Autodesk Fusion 360 part; units mm, degrees
note: some values were not read from the file. Chosen so that the rebuilt part matches the saved one: which bodies a step acts on; which face or edge a step refers to. Set by a fixed rule: which sketch regions a step uses.
(part 4 of 4)
sketch "Base" plane through (0, 0, 52) normal (0, 0, 1) x (-1, 0, 0) in component "GPS"
  circle A0 centre (42.25, -34) radius 1.5
  circle A1 centre (-28.4, 34) radius 1.5
  circle A2 centre (-69.85, 16) radius 1.5
  arc A3 (32.5282, -1.6218) -> (32.5282, 1.6218) centre (30.9065, 0) ccw
  line L0 (32.5282, -1.6218) -> (14.9, -19.25)
  line L1 (14.9, -19.25) -> (7.5026, -19.25)
  arc A4 (5.6636, -14.8105) -> (7.5026, -19.25) centre (7.5026, -16.6494) ccw
  line L2 (5.6636, -14.8105) -> (18.5125, -1.9617)
  arc A5 (18.5125, -1.9617) -> (18.5125, 1.9617) centre (16.5508, 0) ccw
  line L3 (18.5125, 1.9617) -> (5.6636, 14.8105)
  arc A6 (7.5026, 19.25) -> (5.6636, 14.8105) centre (7.5026, 16.6494) ccw
  line L4 (7.5026, 19.25) -> (14.9, 19.25)
  line L5 (14.9, 19.25) -> (32.5282, 1.6218)
  circle A7 centre (-37.85, 16) radius 1.5
  arc A8 (3.4193, -1.5227) -> (3.4193, 1.5227) centre (1.8966, 0) ccw
  line L6 (3.4193, -1.5227) -> (-13.4941, -18.4361)
  spline S0 degree 5 poles (-13.4941, -18.4361) (-13.5655, -18.5075) (-13.7132, -18.651) (-13.9496, -18.869) (-14.3035, -19.15) (-14.8512, -19.4045) (-15.5396, -19.4698) (-16.3722, -19.2715) (-17.2898, -18.7896) (-18.1939, -18.0372) (-18.9671, -17.0431) (-19.3888, -16.0795) (-19.5532, -15.2733) (-19.5897, -14.7) (-19.5897, -14.4044) knots 0 0 0 0 0 0 0.1 0.2 0.3 0.4 0.5 0.6 0.7 0.8 0.9 1 1 1 1 1 1
  line L7 (-19.5897, -14.4044) -> (-19.5897, 14.4044)
  spline S1 degree 5 poles (-19.5897, 14.4044) (-19.5897, 14.7) (-19.5532, 15.2733) (-19.3888, 16.0795) (-18.9671, 17.0431) (-18.1939, 18.0372) (-17.2898, 18.7896) (-16.3722, 19.2715) (-15.5396, 19.4698) (-14.8512, 19.4045) (-14.3035, 19.15) (-13.9496, 18.869) (-13.7132, 18.651) (-13.5655, 18.5075) (-13.4941, 18.4361) knots -1 -1 -1 -1 -1 -1 -0.9 -0.8 -0.7 -0.6 -0.5 -0.4 -0.3 -0.2 -0.1 0 0 0 0 0 0
  line L8 (-13.4941, 18.4361) -> (3.4193, 1.5227)
  circle A9 centre (-28.4, -34) radius 1.5
  circle A10 centre (50.25, -29.25) radius 4
  circle A11 centre (-37.85, -16) radius 1.5
  circle A12 centre (-69.85, -16) radius 1.5
  line L9 (-8, -24.75) -> (24.8, -24.75)
  line L10 (24.8, -24.75) -> (27.0868, -27.0368)
  arc A13 (26.2737, -29) -> (27.0868, -27.0368) centre (26.2737, -27.85) ccw
  line L11 (26.2737, -29) -> (-9.4737, -29)
  arc A14 (-10.2868, -27.0368) -> (-9.4737, -29) centre (-9.4737, -27.85) ccw
  line L12 (-10.2868, -27.0368) -> (-8, -24.75)
  line L13 (27.0868, 27.0368) -> (24.8, 24.75)
  line L14 (24.8, 24.75) -> (-8, 24.75)
  line L15 (-8, 24.75) -> (-10.2868, 27.0368)
  arc A15 (-9.4737, 29) -> (-10.2868, 27.0368) centre (-9.4737, 27.85) ccw
  line L16 (-9.4737, 29) -> (26.2737, 29)
  arc A16 (27.0868, 27.0368) -> (26.2737, 29) centre (26.2737, 27.85) ccw
  line L17 (56.2, 11.1318) -> (56.2, -11.1318)
  arc A17 (55.4036, -12.729) -> (56.2, -11.1318) centre (54.2, -11.1318) ccw
  line L18 (55.4036, -12.729) -> (46.75, -19.25)
  line L19 (46.75, -19.25) -> (36.9216, -19.25)
  arc A18 (34.9726, -14.5445) -> (36.9216, -19.25) centre (36.9216, -16.4936) ccw
  line L20 (34.9726, -14.5445) -> (47.8662, -1.6509)
  arc A19 (47.8662, -1.6509) -> (47.8662, 1.6509) centre (46.2153, 0) ccw
  line L21 (47.8662, 1.6509) -> (34.9726, 14.5445)
  arc A20 (36.9216, 19.25) -> (34.9726, 14.5445) centre (36.9216, 16.4936) ccw
  line L22 (36.9216, 19.25) -> (46.75, 19.25)
  line L23 (46.75, 19.25) -> (55.4036, 12.729)
  arc A21 (56.2, 11.1318) -> (55.4036, 12.729) centre (54.2, 11.1318) ccw
  circle A22 centre (42.25, 34) radius 1.5
  line L24 (70.5, -12.5) -> (70.5, 12.5)
  line L25 (70.5, 12.5) -> (54.7221, 33.4587)
  arc A23 (54.7221, 33.4587) -> (52.2059, 35.2279) centre (50.7275, 30.4515) ccw
  line L26 (52.2059, 35.2279) -> (43.25, 38)
  line L27 (43.25, 38) -> (31.65, 38)
  line L28 (31.65, 38) -> (27.15, 33.5)
  line L29 (27.15, 33.5) -> (-9.25, 33.5)
  line L30 (-9.25, 33.5) -> (-13.75, 38)
  line L31 (-13.75, 38) -> (-30, 38)
  line L32 (-30, 38) -> (-42, 26.25)
  line L33 (-42, 26.25) -> (-70.822, 21.4463)
  arc A24 (-70.822, 21.4463) -> (-75, 16.5144) centre (-70, 16.5144) ccw
  line L34 (-75, 16.5144) -> (-75, -16.5144)
  arc A25 (-75, -16.5144) -> (-70.822, -21.4463) centre (-70, -16.5144) ccw
  line L35 (-70.822, -21.4463) -> (-42, -26.25)
  line L36 (-42, -26.25) -> (-30, -38)
  line L37 (-30, -38) -> (-13.75, -38)
  line L38 (-13.75, -38) -> (-9.25, -33.5)
  line L39 (-9.25, -33.5) -> (27.15, -33.5)
  line L40 (27.15, -33.5) -> (31.65, -38)
  line L41 (31.65, -38) -> (43.25, -38)
  line L42 (43.25, -38) -> (52.2059, -35.2279)
  arc A26 (52.2059, -35.2279) -> (54.7221, -33.4587) centre (50.7275, -30.4515) ccw
  line L43 (54.7221, -33.4587) -> (70.5, -12.5)
  line L44 (-37.85, -16) -> (-69.85, 16) construction
  line L45 (-69.85, -16) -> (-37.85, 16) construction
  arc A27 (-44.4808, -13.9654) -> (-39.8846, -9.3692) centre (-42.1827, -11.6673) ccw
  arc A28 (-67.8154, -9.3692) -> (-63.2192, -13.9654) centre (-65.5173, -11.6673) ccw
  arc A29 (-63.2192, 13.9654) -> (-67.8154, 9.3692) centre (-65.5173, 11.6673) ccw
  arc A30 (-39.8846, 9.3692) -> (-44.4808, 13.9654) centre (-42.1827, 11.6673) ccw
  line L46 (-66.5779, -10.6066) -> (-61.9817, -6.0104)
  line L47 (-64.4566, -12.7279) -> (-59.8604, -8.1317)
  arc A31 (-59.8604, -8.1317) -> (-61.9817, -6.0104) centre (-60.9211, -7.0711) ccw
  arc A32 (-66.5779, -10.6066) -> (-64.4566, -12.7279) centre (-65.5173, -11.6673) ccw
  line L48 (-41.1221, -10.6066) -> (-45.7183, -6.0104)
  arc A33 (-43.2434, -12.7279) -> (-41.1221, -10.6066) centre (-42.1827, -11.6673) ccw
  line L49 (-43.2434, -12.7279) -> (-47.8396, -8.1317)
  arc A34 (-45.7183, -6.0104) -> (-47.8396, -8.1317) centre (-46.7789, -7.0711) ccw
  line L50 (-43.2434, 12.7279) -> (-47.8396, 8.1317)
  arc A35 (-41.1221, 10.6066) -> (-43.2434, 12.7279) centre (-42.1827, 11.6673) ccw
  line L51 (-41.1221, 10.6066) -> (-45.7183, 6.0104)
  arc A36 (-47.8396, 8.1317) -> (-45.7183, 6.0104) centre (-46.7789, 7.0711) ccw
  line L52 (-66.5779, 10.6066) -> (-61.9817, 6.0104)
  arc A37 (-64.4566, 12.7279) -> (-66.5779, 10.6066) centre (-65.5173, 11.6673) ccw
  line L53 (-64.4566, 12.7279) -> (-59.8604, 8.1317)
  arc A38 (-61.9817, 6.0104) -> (-59.8604, 8.1317) centre (-60.9211, 7.0711) ccw
  arc A39 (-58.2391, -8.9853) -> (-49.4609, -8.9853) centre (-53.85, 0) ccw
  arc A40 (-44.8647, -4.3891) -> (-44.8647, 4.3891) centre (-53.85, 0) ccw
  arc A41 (-49.4609, 8.9853) -> (-58.2391, 8.9853) centre (-53.85, 0) ccw
  arc A42 (-62.8353, 4.3891) -> (-62.8353, -4.3891) centre (-53.85, 0) ccw
  line L54 (-44.4808, -13.9654) -> (-49.4609, -8.9853)
  line L55 (-44.8647, -4.3891) -> (-39.8846, -9.3692)
  line L56 (-63.2192, -13.9654) -> (-58.2391, -8.9853)
  line L57 (-44.8647, 4.3891) -> (-39.8846, 9.3692)
  line L58 (-49.4609, 8.9853) -> (-44.4808, 13.9654)
  line L59 (-63.2192, 13.9654) -> (-58.2391, 8.9853)
  line L60 (-62.8353, 4.3891) -> (-67.8154, 9.3692)
  line L61 (-67.8154, -9.3692) -> (-62.8353, -4.3891)
  dimension "d383" = 20
  dimension "d384" = 6.5
  dimension "d385" = 6.5
  dimension "d386" = 6.5
  dimension "d387" = 6.5
  dimension "d388" = 33
  dimension "d389" = 33
  dimension "d390" = 16.5
  dimension "d391" = 16.5
  dimension "d392" = 3
  dimension "d393" = 3
  dimension "d394" = 6.5
  dimension "d396" = 360
  constraint coincident A11.centre L44.start
  constraint coincident A2.centre L44.end
  constraint coincident A12.centre L45.start
  constraint coincident A7.centre L45.end
  constraint midpoint L45 A39.centre
  constraint coincident L45 A28.centre
  constraint coincident L45 A30.centre
  constraint coincident L44 A27.centre
  constraint coincident L44 A29.centre
  constraint tangent A30 L56
  constraint tangent A30 L61
  constraint tangent A29 L54
  constraint tangent A27 L59
  constraint parallel L44 L54
  constraint parallel L44 L59
  constraint parallel L45 L56
  constraint parallel L45 L61
  constraint concentric A28 A32
  constraint coincident L45 A31.centre
  constraint tangent L46 A31
  constraint tangent L47 A31
  constraint parallel L45 L47
  constraint parallel L45 L46
  constraint concentric A39 A40
  constraint coincident A40.start L59
  constraint coincident A40.end L56
  constraint concentric A40 A41
  constraint concentric A41 A42
  constraint coincident A42.start L54
  constraint equal A39 A40
  constraint equal A41 A42
  constraint equal A39 A41
  constraint collinear L55 L59
  constraint collinear L56 L57
  constraint collinear L58 L61
  constraint tangent A29 L60
  measures "d383" diameter of A39
  measures "d384" diameter of A28
  measures "d385" diameter of A30
  measures "d386" diameter of A27
  measures "d387" diameter of A29
  measures "d388" distance of A28.centre A30.centre
  measures "d389" distance of A27.centre A29.centre
  measures "d390" distance of A39.centre A29.centre
  measures "d391" distance of A39.centre A28.centre
  measures "d392" diameter of A32
  measures "d393" diameter of A31
  measures "d394" distance of A28.centre A31.centre
extrude "Extrude1'''''''" add sketch "Base" along normal blind 2.5 separate body contours A27 A28 A29 A30 A39 A40 A41 A42 L54 L55 L56 L57 L58 L59 L60 L61 makes body 58 in component "GPS"
sketch "Sketch2 (2)" plane through (0, 0, 54.5) normal (0, 0, 1) x (-1, 0, 0) in component "GPS"
  arc A0 (-41.1221, 10.6066) -> (-43.2434, 12.7279) centre (-42.1827, 11.6673) ccw
  line L0 (-41.1221, 10.6066) -> (-45.7183, 6.0104)
  arc A1 (-47.8396, 8.1317) -> (-45.7183, 6.0104) centre (-46.7789, 7.0711) ccw
  line L1 (-47.8396, 8.1317) -> (-43.2434, 12.7279)
  arc A2 (-43.2434, -12.7279) -> (-41.1221, -10.6066) centre (-42.1827, -11.6673) ccw
  line L2 (-43.2434, -12.7279) -> (-47.8396, -8.1317)
  arc A3 (-45.7183, -6.0104) -> (-47.8396, -8.1317) centre (-46.7789, -7.0711) ccw
  line L3 (-45.7183, -6.0104) -> (-41.1221, -10.6066)
  arc A4 (-66.5779, -10.6066) -> (-64.4566, -12.7279) centre (-65.5173, -11.6673) ccw
  line L4 (-66.5779, -10.6066) -> (-61.9817, -6.0104)
  arc A5 (-59.8604, -8.1317) -> (-61.9817, -6.0104) centre (-60.9211, -7.0711) ccw
  line L5 (-59.8604, -8.1317) -> (-64.4566, -12.7279)
  arc A6 (-64.4566, 12.7279) -> (-66.5779, 10.6066) centre (-65.5173, 11.6673) ccw
  line L6 (-64.4566, 12.7279) -> (-59.8604, 8.1317)
  arc A7 (-61.9817, 6.0104) -> (-59.8604, 8.1317) centre (-60.9211, 7.0711) ccw
  line L7 (-61.9817, 6.0104) -> (-66.5779, 10.6066)
  line L8 (-63.2192, -13.9654) -> (-58.2391, -8.9853)
  arc A8 (-58.2391, -8.9853) -> (-49.4609, -8.9853) centre (-53.85, 0) ccw
  line L9 (-49.4609, -8.9853) -> (-44.4808, -13.9654)
  arc A9 (-44.4808, -13.9654) -> (-39.8846, -9.3692) centre (-42.1827, -11.6673) ccw
  line L10 (-39.8846, -9.3692) -> (-44.8647, -4.3891)
  arc A10 (-44.8647, -4.3891) -> (-44.8647, 4.3891) centre (-53.85, 0) ccw
  line L11 (-44.8647, 4.3891) -> (-39.8846, 9.3692)
  arc A11 (-39.8846, 9.3692) -> (-44.4808, 13.9654) centre (-42.1827, 11.6673) ccw
  line L12 (-44.4808, 13.9654) -> (-49.4609, 8.9853)
  arc A12 (-49.4609, 8.9853) -> (-58.2391, 8.9853) centre (-53.85, 0) ccw
  line L13 (-58.2391, 8.9853) -> (-63.2192, 13.9654)
  arc A13 (-63.2192, 13.9654) -> (-67.8154, 9.3692) centre (-65.5173, 11.6673) ccw
  line L14 (-67.8154, 9.3692) -> (-62.8353, 4.3891)
  arc A14 (-62.8353, 4.3891) -> (-62.8353, -4.3891) centre (-53.85, 0) ccw
  line L15 (-62.8353, -4.3891) -> (-67.8154, -9.3692)
  arc A15 (-67.8154, -9.3692) -> (-63.2192, -13.9654) centre (-65.5173, -11.6673) ccw
  circle A16 centre (-53.85, 0) radius 7.575
  dimension "d399" = 15.15
  constraint concentric A8 A16
  measures "d399" diameter of A16
extrude "Extrude2'''''''" add sketch "Sketch2 (2)" along normal blind 13 contours A16 bodies 58 in component "GPS"
extrude "Extrude3'" add 1 faces at (57.0866, -1.5086, 67.5) along direction (0, 0, 1) blind 14.5 draft -12 on bodies 58 bodies 58 in component "GPS"
sketch "Sketch3" plane through (0, 0, 82) normal (0, 0, 1) x (-1, 0, 0) in component "GPS"
  circle A0 centre (-53.85, 0) radius 4.4929
  circle A1 centre (-53.85, 0) radius 1.95
  dimension "d404" = 3.9
  constraint concentric A0 A1
  measures "d404" diameter of A1
extrude "Extrude4'" add sketch "Sketch3" along normal blind 130 contours A1 bodies 58 in component "GPS"
sketch "GPS Mount" plane through (0, 0, 212) normal (0, 0, 1) x (-1, 0, 0) in component "GPS"
  circle A0 centre (-53.85, 0) radius 1.95
  circle A1 centre (-53.85, 0) radius 17.375
  circle A2 centre (-53.85, 0) radius 7.5
  dimension "d407" = 34.75
  dimension "d410" = 15
  constraint concentric A0 A1
  constraint concentric A1 A2
  measures "d407" diameter of A1
  measures "d410" diameter of A2
extrude "Extrude5'" add sketch "GPS Mount" along normal blind 1.5 contours A0 | A1 | A2 bodies 58 in component "GPS"
extrude "Extrude6'" add sketch "GPS Mount" against normal blind 10 draft -25 contours A2 bodies 58 in component "GPS"
component "Bottom Plate" placed x (1, 0, 0) y (0, 1, 0) z (0, 0, 1) at (0, 0, 0)
component "Top Plate" placed x (1, 0, 0) y (0, 1, 0) z (0, 0, 1) at (0, 0, 0)
component "Pixhawk Plate" placed x (1, 0, 0) y (0, 1, 0) z (0, 0, 1) at (0, 0, 0)
component "Accessory Plate" placed x (1, 0, 0) y (0, 1, 0) z (0, 0, 1) at (0, 0, 0)
component "Arm NW" placed x (1, 0, 0) y (0, 1, 0) z (0, 0, 1) at (0, 0, 0)
component "Arm NE (Mirror)" placed x (-1, 0, 0) y (0, 1, 0) z (0, 0, -1) at (-22.5, 0, 0)
component "Arm SW (Mirror 2)" placed x (1, 0, 0) y (0, -1, 0) z (0, 0, -1) at (0, 0, 0)
component "Arm SE (Mirror 2)" placed x (-1, 0, 0) y (0, -1, 0) z (0, 0, 1) at (-22.5, 0, 0)
component "GPS" placed x (1, 0, 0) y (0, 1, 0) z (0, 0, 1) at (0, 0, 0)
component "Leg NW" placed x (1, 0, 0) y (0, 1, 0) z (0, 0, 1) at (0, 0, 0) in component "Arm NW"
component "Motor Plate" placed x (1, 0, 0) y (0, 1, 0) z (0, 0, 1) at (0, 0, 0) in component "Arm NW"
component "Motor" placed x (1, 0, 0) y (0, 1, 0) z (0, 0, 1) at (0, 0, 0) in component "Arm NW"
component "Leg NW(Mirror)" placed x (1, 0, 0) y (0, 1, 0) z (0, 0, 1) at (0, 0, 0) in component "Arm NE (Mirror)"
component "Motor Plate(Mirror)" placed x (1, 0, 0) y (0, 1, 0) z (0, 0, 1) at (0, 0, 0) in component "Arm NE (Mirror)"
component "Motor(Mirror)" placed x (1, 0, 0) y (0, 1, 0) z (0, 0, 1) at (0, 0, 0) in component "Arm NE (Mirror)"
component "Leg NW(Mirror) (1)" placed x (1, 0, 0) y (0, 1, 0) z (0, 0, 1) at (0, 0, 0) in component "Arm SW (Mirror 2)"
component "Motor Plate(Mirror) (1)" placed x (1, 0, 0) y (0, 1, 0) z (0, 0, 1) at (0, 0, 0) in component "Arm SW (Mirror 2)"
component "Motor(Mirror) (1)" placed x (1, 0, 0) y (0, 1, 0) z (0, 0, 1) at (0, 0, 0) in component "Arm SW (Mirror 2)"
component "Leg NW(Mirror)(Mirror)" placed x (1, 0, 0) y (0, 1, 0) z (0, 0, 1) at (0, 0, 0) in component "Arm SE (Mirror 2)"
component "Motor Plate(Mirror)(Mirror)" placed x (1, 0, 0) y (0, 1, 0) z (0, 0, 1) at (0, 0, 0) in component "Arm SE (Mirror 2)"
component "Motor(Mirror)(Mirror)" placed x (1, 0, 0) y (0, 1, 0) z (0, 0, 1) at (0, 0, 0) in component "Arm SE (Mirror 2)"
hidden bodies 54 55 56 57 32
equation "smale_hole_diameter = 3 mm" comment "Diameter of small holes for bolts."
equation "plate_thickness = 2 mm" comment "Default plate thickness."
equation "arm_length = 240 mm"
equation "arm_width = 19 mm"
equation "d30 = smale_hole_diameter"
equation "d31 = smale_hole_diameter"
equation "d32 = smale_hole_diameter"
equation "d33 = smale_hole_diameter"
equation "d34 = smale_hole_diameter"
equation "d35 = smale_hole_diameter"
equation "d36 = smale_hole_diameter"
equation "d37 = smale_hole_diameter"
equation "d38 = smale_hole_diameter"
equation "d59 = arm_angle"
equation "arm_angle = 117.5 deg"
equation "d61 = arm_angle"
equation "d104 = smale_hole_diameter"
equation "d135 = plate_thickness"
equation "d137 = arm_width"
equation "d138 = arm_width / 2"
equation "d140 = arm_length"
equation "d145 = arm_width"
equation "d148 = -arm_length"
equation "d150 = smale_hole_diameter"
equation "d151 = smale_hole_diameter"
equation "d156 = -arm_width"
equation "d160 = smale_hole_diameter"
equation "d161 = smale_hole_diameter"
equation "d189 = arm_width"
equation "d197 = smale_hole_diameter"
equation "d198 = smale_hole_diameter"
equation "d199 = smale_hole_diameter"
equation "d204 = plate_thickness"
equation "d206 = plate_thickness"
equation "d221 = plate_thickness"
equation "d223 = pixhawk_offset"
equation "d224 = access_offset"
equation "d251 = smale_hole_diameter"
equation "d252 = smale_hole_diameter"
equation "d253 = smale_hole_diameter"
equation "d279 = plate_thickness"
equation "d300 = smale_hole_diameter"
equation "d301 = smale_hole_diameter"
equation "d325 = plate_thickness"
equation "hex_od = 5.5 mm" comment "Hex standoff outer diameter."
equation "collar_od = 6.4 mm" comment "Cylindrical bolt collar outer diameter."
equation "collar_id = 3.4 mm" comment "Cyllindrical bolt collar inner diameter."
equation "d330 = hex_od"
equation "hex_id = 2.5 mm" comment "Approx inner diameter of hex standoff."
equation "d332 = hex_id"
equation "d333 = hex_od"
equation "d334 = hex_id"
equation "d335 = hex_od"
equation "d336 = hex_id"
equation "d337 = -arm_width"
equation "d339 = collar_od"
equation "d340 = collar_id"
equation "d341 = collar_od"
equation "d342 = collar_id"
equation "d343 = collar_od"
equation "d344 = collar_id"
equation "d345 = collar_od"
equation "d346 = collar_id"
equation "d347 = collar_od"
equation "d348 = collar_id"
equation "d349 = collar_od"
equation "d350 = collar_id"
equation "d351 = collar_od"
equation "d352 = collar_id"
equation "d353 = collar_od"
equation "d354 = collar_id"
equation "d355 = -arm_width"
equation "pixhawk_offset = 10 mm" comment "Distance from top plate to Pixhawk plate"
equation "access_offset = 17 mm" comment "Distance from Pixhawk plate to accessory plate"
equation "d359 = hex_od"
equation "d360 = hex_id"
equation "d361 = hex_od"
equation "d362 = hex_id"
equation "d363 = hex_od"
equation "d364 = hex_id"
equation "d365 = hex_od"
equation "d366 = hex_id"
equation "d367 = -pixhawk_offset"
equation "d369 = hex_od"
equation "d370 = hex_id"
equation "d371 = hex_od"
equation "d374 = hex_id"
equation "d376 = hex_od"
equation "d377 = hex_id"
equation "d379 = hex_od"
equation "d380 = hex_id"
equation "d381 = -access_offset + plate_thickness"
equation "d390 = d389 / 2"
equation "d391 = d388 / 2"
equation "d425 = smale_hole_diameter"
equation "d426 = 2.1 mm + smale_hole_diameter / 2"
equation "d427 = smale_hole_diameter"
equation "d428 = 2.1 mm + smale_hole_diameter / 2"
equation "d429 = smale_hole_diameter"
equation "d430 = 2.1 mm + smale_hole_diameter / 2"
equation "d431 = plate_thickness"
named bodies: "Bottom Plate", "Arm NW", "Leg Inner", "Leg Outer", "Top Plate", "Pixhawk Plate", "Accessory Plate", "Hex 1", "Hex 2", "Hex 3", "Collar 1", "Collar 5", "Collar 4", "Collar 8", "Collar 2", "Collar 6", "Collar 3", "Collar 7", "GPS Mast", "Hex 4"
